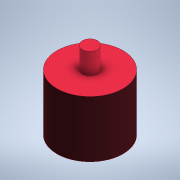
# Autodesk Inventor part: Моторчик
Saved by Autodesk Inventor 2021.2 (Build 252289000, 289)
## iProperties
Created: 2024-10-29
Part Number: Моторчик
Material: Типовые
Document SubType Name: Modeling
Designer: barko
Density: 1 g/cm^3
Appearance: По умолчанию
Author: barko
Autodesk Inventor part; units mm, degrees
ref_plane "YZ Plane" through (0, 0, 0) normal (1, 0, 0) x (0, 1, 0)
ref_plane "XZ Plane" through (0, 0, 0) normal (0, 1, 0) x (-1, 0, 0)
ref_plane "XY Plane" through (0, 0, 0) normal (0, 0, 1) x (1, 0, 0)
sketch "Эскиз1" plane through (0, 0, 0) normal (0, 0, 1) x (1, 0, 0)
  line L0 (0, 0) -> (0, 33)
  line L1 (0, 0) -> (-14, 0)
  line L2 (-14, 0) -> (-14, 24)
  line L3 (-14, 24) -> (-3.25, 24)
  line L4 (-3.25, 24) -> (-3.25, 33)
  line L5 (-3.25, 33) -> (0, 33)
  dimension "d0" = 24
  dimension "d1" = 28
  dimension "d2" = 6.5
  dimension "d3" = 9
  constraints: 13 end point, 3 perpendicular, 1 horizontal, 1 parallel, 1 vertical
  measures "d0" distance between parallel lines of L3 L1
  measures "d1" diameter of L2 L0
  measures "d2" diameter of L4 L0
  measures "d3" distance between parallel lines of L3 L5
revolve "Вращение1" add sketch "Эскиз1" angle 360 about axis through (0, 0, 0) along (0, 1, 0)
equation "\"d0\" = motor_height"
equation "\"d1\" = motor_diameter"
equation "\"blade_radius\" = 127"
equation "\"bearing_inner\" = 7"
equation "\"bearing_outer\" = 19"
equation "\"bearing_width\" = 6"
equation "\"beam_length\" = 254"
equation "\"motor_height\" = 24"
equation "\"motor_diameter\" = 28"
equation "\"motor_blade_offset\" = 2"
